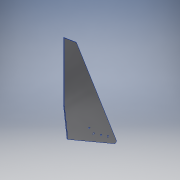
# Autodesk Inventor part: stay_middle
Saved by Autodesk Inventor 2018.1 (Build 221171000, 171)
## iProperties
Created: 2017-10-18
Part Number: stay_middle
Material: アルミニウム 6061
Document SubType Name: Modeling
Designer: kuwano
Density: 2.7 g/cm^3
Appearance: アルミニウム - フラット
Mass: 236.173 g
Surface Area: 610.603 cm^2
Volume: 87.4716 cm^3
Author: kuwano
Autodesk Inventor part; units mm, degrees
ref_plane "YZ Plane" through (0, 0, 0) normal (1, 0, 0) x (0, 1, 0)
ref_plane "XZ Plane" through (0, 0, 0) normal (0, 1, 0) x (-1, 0, 0)
ref_plane "XY Plane" through (0, 0, 0) normal (0, 0, 1) x (1, 0, 0)
sketch "スケッチ1" plane through (0, 0, 0) normal (1, 0, 0) x (0, 1, 0)
  line L0 (-90, 100) -> (-90, -100)
  line L1 (-90, -100) -> (-78.3609, -202.4286)
  line L2 (-78.3609, -202.4286) -> (90, -300)
  line L3 (-126, 0) -> (126, 0) projected
  line L4 (0, -380) -> (0, 180) projected
  line L5 (-90, 100) -> (-49.5962, 66.2658)
  line L6 (-49.5962, 66.2658) -> (90, -300)
  point P0 (-90, 0)
  dimension "d0" = 200
  dimension "d5" = 90
  dimension "d6" = 300
  dimension "d7" = 90
  constraints: 10 end point, 1 midpoint, 1 point on line, 1 vertical
  measures "d0" distance of L0.start L0.end
  measures "d5" distance between parallel lines of L0 L4
  measures "d6" distance from line of L3 L2.end
  measures "d7" distance from line of L4 L2.end
extrude "押し出し1" add sketch "スケッチ1" along normal blind 3 contours L5 L6 L3 L0 | L3 L6 L4 L2 L1 L0 | L6 L2 L4
fillet "フィレット1" radius 5 1 edges at (1.5, 90, -300)
sketch "スケッチ2" plane through (0, 0, 0) normal (-1, 0, 0) x (0, 0, 1)
  circle A0 centre (-261.0423, 56.959) radius 2.5
  line L0 (-286.8218, 84.9773) -> (66.2658, -49.5962) projected
  line L1 (-202.4286, -78.3609) -> (-292.9285, 77.7981) projected
  circle A1 centre (-245.5451, 33.9298) radius 2.5
  circle A2 centre (-204.9844, -6.1431) radius 2.5
  circle A3 centre (-228.7174, 8.2532) radius 2.5
  circle A4 centre (-89.8899, -23.2553) radius 2.5
  circle A5 centre (-175.3487, -22.7892) radius 2.5
  point P0 (0, 0)
  dimension "d10" = 5
  dimension "d11" = 19
  dimension "d12" = 33
  dimension "d13" = 5
  dimension "d14" = 27.758
  dimension "d15" = 17
  dimension "d16" = 56
  dimension "d17" = 34
  dimension "d18" = 27.758
  dimension "d19" = 5
  dimension "d20" = 5
  dimension "d21" = 51
  dimension "d24" = 31
  dimension "d25" = 5
  dimension "d26" = 125
  dimension "d27" = 85.46
  dimension "d28" = 5
  dimension "d29" = 61
  constraints: 6 centre point
  measures "d10" diameter of A0
  measures "d11" distance from line of L1 A1.centre
  measures "d12" distance from line of L0 A1.centre
  measures "d13" diameter of A1
  measures "d14" distance of A1.centre A0.centre
  measures "d15" distance from line of L0 A0.centre
  measures "d16" distance from line of L0 A2.centre
  measures "d17" distance from line of L1 A2.centre
  measures "d18" distance of A2.centre A3.centre
  measures "d19" diameter of A3
  measures "d20" diameter of A2
  measures "d21" distance from line of L0 A3.centre
  measures "d24" distance from line of L0 A4.centre
  measures "d25" diameter of A4
  measures "d26" distance from line of L1 A4.centre
  measures "d27" distance of A4.centre A5.centre
  measures "d28" diameter of A5
  measures "d29" distance from line of L0 A5.centre
extrude "押し出し2" cut sketch "スケッチ2" against normal up to next
